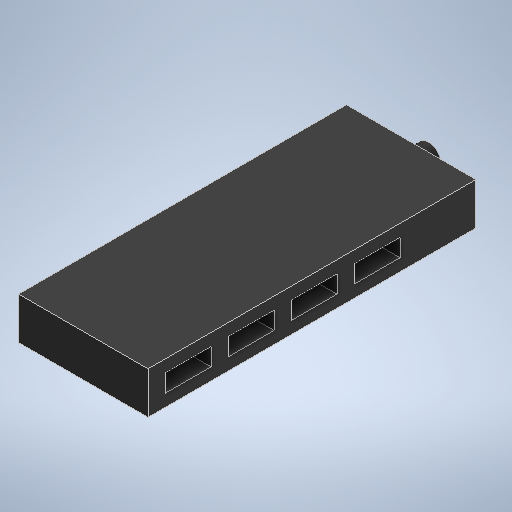
# Autodesk Inventor part: USBextender
Saved by Autodesk Inventor 2025.2 (Build 292293000, 293)
## iProperties
Created: 2025-08-10
Part Number: USBextender
Material: Generic
Document SubType Name: Modeling
Designer: hofma
Density: 1 g/cm^3
Appearance: Default(1)
Author: hofma
Autodesk Inventor part; units mm, degrees
ref_plane "YZ Plane" through (0, 0, 0) normal (1, 0, 0) x (0, 1, 0)
ref_plane "XZ Plane" through (0, 0, 0) normal (0, 1, 0) x (-1, 0, 0)
ref_plane "XY Plane" through (0, 0, 0) normal (0, 0, 1) x (1, 0, 0)
sketch "Sketch1" plane through (0, 0, 0) normal (0, 1, 0) x (-1, 0, 0)
  line L0 (18.5, 46.85) -> (-18.5, 46.85)
  line L1 (-18.5, 46.85) -> (-18.5, -46.85)
  line L2 (-18.5, -46.85) -> (18.5, -46.85)
  line L3 (18.5, -46.85) -> (18.5, 46.85)
  line L4 (18.5, 46.85) -> (-18.5, -46.85) construction
  line L5 (-18.5, 46.85) -> (18.5, -46.85) construction
  point P0 (0, 0)
  dimension "d0" = 93.7
  dimension "d1" = 37
  constraints: 12 end point, 2 midpoint, 2 parallel, 1 horizontal, 1 perpendicular
  measures "d0" distance of L2.end L0.start
  measures "d1" distance of L0.start L0.end
extrude "Extrusion1" add sketch "Sketch1" along normal blind 12
sketch "Sketch2" plane through (18.5, 0, 46.85) normal (1, 0, 0) x (0, 0, -1)
  line L0 (5, 3.5) -> (18, 3.5)
  line L1 (18, 3.5) -> (18, 8.5)
  line L2 (18, 8.5) -> (5, 8.5)
  line L3 (5, 8.5) -> (5, 3.5)
  line L4 (5, 3.5) -> (18, 8.5) construction
  line L5 (18, 3.5) -> (5, 8.5) construction
  line L6 (23, 3.5) -> (36, 3.5)
  line L7 (36, 3.5) -> (36, 8.5)
  line L8 (36, 8.5) -> (23, 8.5)
  line L9 (23, 8.5) -> (23, 3.5)
  line L10 (23, 3.5) -> (36, 8.5) construction
  line L11 (36, 3.5) -> (23, 8.5) construction
  line L12 (41, 3.5) -> (54, 3.5)
  line L13 (54, 3.5) -> (54, 8.5)
  line L14 (54, 8.5) -> (41, 8.5)
  line L15 (41, 8.5) -> (41, 3.5)
  line L16 (41, 3.5) -> (54, 8.5) construction
  line L17 (54, 3.5) -> (41, 8.5) construction
  line L18 (59, 3.5) -> (72, 3.5)
  line L19 (72, 3.5) -> (72, 8.5)
  line L20 (72, 8.5) -> (59, 8.5)
  line L21 (59, 8.5) -> (59, 3.5)
  line L22 (59, 3.5) -> (72, 8.5) construction
  line L23 (72, 3.5) -> (59, 8.5) construction
  line L24 (0, 0) -> (0, 12) projected
  point P0 (46.85, 0)
  point P1 (11.5, 6)
  point P2 (29.5, 6)
  point P3 (47.5, 6)
  point P4 (65.5, 6)
  point P5 (0, 6)
  point P6 (54, 6)
  dimension "d4" = 5
  dimension "d5" = 5
  dimension "d6" = 5
  dimension "d7" = 5
  dimension "d8" = 13
  dimension "d9" = 5
  constraints: 48 end point, 10 midpoint, 8 parallel, 6 equal length, 4 horizontal, 4 horizontal alignment, 4 perpendicular
  measures "d4" distance between parallel lines of L3 L24
  measures "d5" distance between parallel lines of L9 L1
  measures "d6" distance between parallel lines of L15 L7
  measures "d7" distance from line of L21 point (54, 6)
  measures "d8" distance of L1.end L2.end
  measures "d9" distance between parallel lines of L0 L2
extrude "Extrusion2" cut sketch "Sketch2" against normal blind 12
sketch "Sketch3" plane through (18.5, 0, -46.85) normal (0, 0, -1) x (-1, 0, 0)
  circle A0 centre (18.5, 6) radius 3.5
  point P0 (18.5, 0)
  dimension "d12" = 7
  constraints: 1 centre point
  measures "d12" diameter of A0
extrude "Extrusion3" add sketch "Sketch3" along normal blind 5
equation "\"d5\" = d4"
equation "\"d6\" = d5"
equation "\"d7\" = d6"
body "Solid1"
